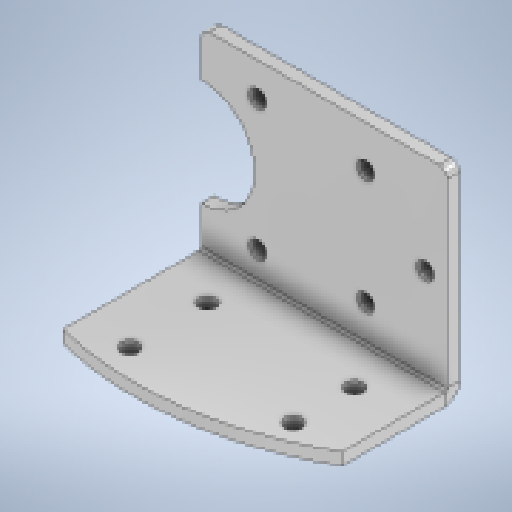
# Autodesk Inventor part: axis_2_bottom_L_frame(top)
Saved by Autodesk Inventor 2024.2 (Build 282272000, 272)
## iProperties
Created: 2023-09-15
Part Number: axis_2_bottom_L_frame(top)
Material: Aluminum 6061-AHC
Document SubType Name: Sheet Metal
Designer: chanh
Density: 2.7 g/cm^3
Sheet Metal Rule: Default_mm
Appearance: Aluminum - Dark
Author: chanh
Autodesk Inventor part; units mm, degrees
ref_plane "YZ Plane" through (0, 0, 0) normal (1, 0, 0) x (0, 1, 0)
ref_plane "XZ Plane" through (0, 0, 0) normal (0, 1, 0) x (-1, 0, 0)
ref_plane "XY Plane" through (0, 0, 0) normal (0, 0, 1) x (1, 0, 0)
sketch "Sketch1" plane through (0, 0, 0) normal (0, 0, 1) x (1, 0, 0)
  line L0 (-15.05, -12.5) -> (15.05, -12.5)
  line L1 (15.05, -12.5) -> (15.05, 12.5)
  line L2 (15.05, 12.5) -> (-15.05, 12.5)
  line L3 (-15.05, 12.5) -> (-15.05, -12.5)
  line L4 (-15.05, -12.5) -> (15.05, 12.5) construction
  line L5 (15.05, -12.5) -> (-15.05, 12.5) construction
  point P0 (0, 0)
  dimension "d0" = 30.1
  dimension "d1" = 25
  measures "d0" distance of L2.end L1.end
  measures "d1" distance of L1.end L0.end
extrude "Plate1" add sketch "Sketch1" along normal blind 1.5
sketch "Sketch6" plane through (0, 0, 1.5) normal (0, 0, 1) x (1, 0, 0)
  circle A0 centre (-8.15, 9.43) radius 0.7835 projected
  circle A1 centre (-8.15, -6.57) radius 0.7835 projected
  circle A2 centre (5.07, 8.43) radius 0.7835 projected
  circle A3 centre (5.07, -5.57) radius 0.7835 projected
  circle A4 centre (12.37, 1.43) radius 0.7835 projected
  point P0 (0, 0)
hole "Hole2" at (-8.15, 9.43, 1.5) at (5.07, 8.43, 1.5) at (12.37, 1.43, 1.5) at (5.07, -5.57, 1.5) at (-8.15, -6.57, 1.5) direction (0, 0, -1) diameter 2.1 end through all
sketch "Sketch7" plane through (0, 0, 1.5) normal (0, 0, 1) x (1, 0, 0)
  circle A0 centre (-15.05, 1.43) radius 6.4 projected
  circle A1 centre (-15.05, 1.43) radius 6.55
  point P0 (0, 0)
  dimension "d42" = 0.15
  constraints: 1 centre point, 1 coincident
  measures "d42" radial gap between concentric circles of A1 A0
extrude "Cut1" cut sketch "Sketch7" against normal blind 1.5 contours A0 | A1
sketch "Sketch8" plane through (15.05, -11, 0) normal (0, -1, 0) x (1, 0, 0)
  line L0 (-30.1, 0) -> (0, 0)
  line L1 (0, 0) -> (0, 20)
  line L2 (0, 20) -> (-30.1, 20)
  line L3 (-30.1, 20) -> (-30.1, 0)
  constraints: 6 end point, 1 horizontal, 1 perpendicular, 1 vertical
edge flange "Flange2" height 20 angle 90 thickness 1.5 bend radius 0.31 thickness toward (0, -1, 0) relief tear relief width 1.5 relief depth 0.75 edges at (0, -12.5, 1.5) wall of the first edge with corners at (-15.05, -11, 0) (15.05, -11, 0) (15.05, -11, 20) (-15.05, -11, 20)
bend "Bend2"
corner "Corner2"
sketch "Sketch9" plane through (-15.05, -11, 20) normal (0, 1, 0) x (1, 0, 0)
  circle A0 centre (10.05, 40.25) radius 40 projected
  circle A1 centre (10.05, 40.25) radius 50
  point P0 (15.05, 20)
  dimension "d39" = 10
  constraints: 1 centre point, 1 coincident
  measures "d39" radial gap between concentric circles of A1 A0
extrude "Cut2" cut sketch "Sketch9" against normal blind 1.5
fillet "Corner Round1" radius 1 2 edges at (15.05, 12.5, 0.75) (-15.05, 12.5, 0.75)
sketch "Sketch10" plane through (-15.05, -11, 1.81) normal (0, 1, 0) x (1, 0, 0)
  line L0 (30.1, 0) -> (0, 0) projected
  arc A0 (0, -16.6569) -> (30.1, -12.5521) centre (10.05, 22.06) ccw projected
  line L1 (15.05, 0) -> (15.05, -17.6263) construction
  point P0 (15.05, 1.81)
  point P1 (6.05, -5)
  point P2 (24.05, -5)
  point P3 (24.05, -12.5)
  point P4 (6.05, -14.5)
  dimension "d44" = 18
  dimension "d45" = 9.5
  dimension "d46" = 7.5
  dimension "d47" = 5
  constraints: 2 end point, 2 vertical alignment, 1 horizontal alignment, 1 midpoint, 1 point on circle, 1 symmetric about line, 1 vertical
  measures "d44" distance of point (24.05, -5) point (6.05, -5)
  measures "d45" distance of point (6.05, -14.5) point (6.05, -5)
  measures "d46" distance of point (24.05, -5) point (24.05, -12.5)
  measures "d47" distance from line of L0 point (6.05, -5)
hole "Hole3" at (-9, -11, 6.81) at (9, -11, 6.81) at (9, -11, 14.31) at (-9, -11, 16.31) direction (0, -1, 0) diameter 2.1 end through all
equation "\"d27\" = Thickness"
equation "\"d40\" = Thickness"
equation "\"d2\" = Thickness"
equation "\"d29\" = BendReliefWidth"
equation "\"d30\" = BendReliefDepth"
equation "\"d31\" = MinimumRemnant"
equation "\"d32\" = TransitionRadius"
equation "\"d35\" = BendRadius"
equation "\"d36\" = CornerReliefSize"
equation "\"d37\" = GapSize"
equation "\"d38\" = JacobiRadiusSize"
equation "\"BendReliefWidth\" = Thickness"
equation "\"BendReliefDepth\" = 0.5 * Thickness"
equation "\"CornerReliefSize\" = 4 * Thickness"
equation "\"MinimumRemnant\" = 2 * Thickness"
equation "\"TransitionRadius\" = BendRadius"
equation "\"JacobiRadiusSize\" = BendRadius"
equation "\"GapSize\" = Thickness"
equation "\"Thickness\" = 1.5"
equation "\"BendRadius\" = 0.31"
body "Solid1"
